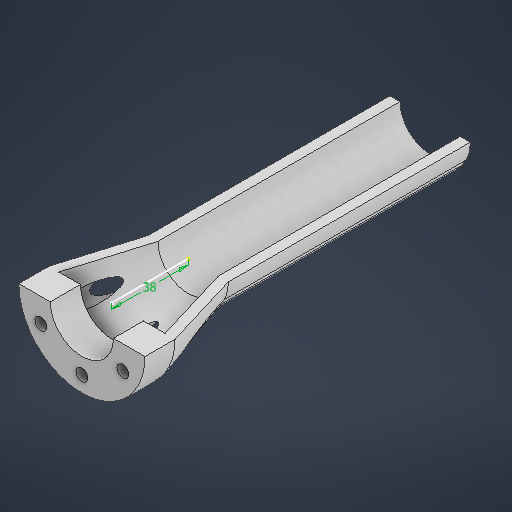
# Autodesk Inventor part: Carcasa_Part1
Saved by Autodesk Inventor 2026.1 (Build 301233020, 233B)
## iProperties
Created: 2026-01-06
Part Number: Carcasa_Part1
Material: Generic
Document SubType Name: Modeling
Designer: Marcelo
Density: 1 g/cm^3
Appearance: Default
Author: Marcelo
Autodesk Inventor part; units mm, degrees
ref_plane "YZ Plane" through (0, 0, 0) normal (1, 0, 0) x (0, 1, 0)
ref_plane "XZ Plane" through (0, 0, 0) normal (0, 1, 0) x (-1, 0, 0)
sketch "Sketch1" plane through (0, 0, 0) normal (0, 0, 1) x (1, 0, 0)
  circle A0 centre (0, 0) radius 20.05
  dimension "d0" = 40.1
  constraints: 1 centre point, 1 coincident
  measures "d0" diameter of A0
extrude "Extrusion1" add sketch "Sketch1" along normal blind 120.75
sketch "Sketch2" plane through (0, 0, 120.75) normal (0, 0, 1) x (1, 0, 0)
  circle A0 centre (0, 0) radius 20.05 projected
  arc A1 (-15.05, 0) -> (15.05, 0) centre (0, 0) ccw
  line L0 (-20.05, 0) -> (20.05, 0)
  dimension "d3" = 5
  constraints: 4 point on circle, 2 end point, 2 horizontal, 2 point on line, 1 centre point
  measures "d3" radial gap between concentric circles of A0 A1
extrude "Extrusion2" cut sketch "Sketch2" against normal blind 120.75 contours L0 A0 | A1 L0
sketch "Sketch3" plane through (0, 0, 120.75) normal (0, 0, 1) x (1, 0, 0)
  point P0 (0, 0)
sketch3d "3D Sketch1"
ref_plane "Work Plane1" through (0, 0, 158.75) normal (0, 0, 1) x (1, 0, 0)
sketch "Sketch4" plane through (0, 0, 158.75) normal (0, 0, 1) x (1, 0, 0)
  circle A0 centre (0, 0) radius 31.5
  circle A1 centre (0, 0) radius 15.75
  dimension "d7" = 63
  dimension "d8" = 31.5
  constraints: 2 centre point, 2 coincident
  measures "d7" diameter of A0
  measures "d8" diameter of A1
extrude "Extrusion3" add sketch "Sketch4" along normal blind 15
sketch "Sketch5" plane through (0, 0, 173.75) normal (0, 0, 1) x (1, 0, 0)
  line L0 (27.2798, -15.75) -> (-27.2798, 15.75)
  line L1 (0, 31.5) -> (0, -31.5)
  circle A0 centre (0, 0) radius 31.5 projected
  line L2 (27.2798, 15.75) -> (-27.2798, -15.75)
  circle A1 centre (0, 0) radius 31.5 projected
  circle A2 centre (0, 0) radius 15.75 projected
  circle A3 centre (0, 0) radius 23.625 construction
  line L3 (0, 0) -> (-31.5, 0) construction
  circle A4 centre (-20.4599, 11.8125) radius 3
  circle A5 centre (0, 23.625) radius 3
  circle A6 centre (20.4599, 11.8125) radius 3
  circle A7 centre (20.4599, -11.8125) radius 3
  circle A8 centre (0, -23.625) radius 3
  circle A9 centre (-20.4599, -11.8125) radius 3
  dimension "d14" = 60
  dimension "d15" = 60
  dimension "d16" = 7.875
  dimension "d17" = 30
  dimension "d18" = 6
  dimension "d19" = 6
  dimension "d20" = 6
  dimension "d21" = 6
  dimension "d22" = 6
  dimension "d23" = 6
  constraints: 11 point on circle, 8 end point, 7 centre point, 6 point on line, 3 midpoint, 1 coincident, 1 horizontal, 2 other
  measures "d14" angle of L1 L0
  measures "d15" angle of L0 L2
  measures "d16" radial gap between concentric circles of A3 A2
  measures "d17" angle of L3 L0
  measures "d18" diameter of A4
  measures "d19" diameter of A5
  measures "d20" diameter of A6
  measures "d21" diameter of A7
  measures "d22" diameter of A8
  measures "d23" diameter of A9
hole "Hole1" at (-20.4599, 11.8125, 173.75) direction (0, 0, -1) diameter 6 end through all
thread "Thread1" size "M6x1" class "6H" standard "ISO Metric profile" full length
pattern_circular "Circular Pattern1" count 6 over 360 about axis through (0, 0, 158.75) along (0, 0, 1) of "Hole1"
sketch "Sketch7" plane through (0, 0, 173.75) normal (0, 0, 1) x (1, 0, 0)
  circle A0 centre (0, 0) radius 31.5 projected
  line L0 (-31.5, 0) -> (31.5, 0)
  constraints: 2 end point, 2 point on circle, 1 horizontal
extrude "Extrusion4" cut sketch "Sketch7" against normal blind 15 contours L0 A0 picked at (9.2973, 4.8796)
sketch "Sketch8" plane through (0, 0, 158.75) normal (0, 0, -1) x (-1, 0, 0)
  arc A0 (-31.5, 0) -> (31.5, 0) centre (0, 0) ccw projected
  arc A1 (-26.5, 0) -> (26.5, 0) centre (0, 0) ccw
  line L0 (-15.75, 0) -> (-31.5, 0) projected
  line L1 (-31.5, 0) -> (-26.5, 0)
  line L2 (26.5, 0) -> (31.5, 0)
  dimension "d39" = 5
  constraints: 4 end point, 2 collinear, 2 point on circle, 1 centre point
  measures "d39" radial gap between concentric circles of A0 A1
loft "Loft1" add profiles "Sketch8" section 1 edges at (-17.55, 0, 120.75) (0, -20.05, 120.75) (17.55, 0, 120.75) (0, -15.05, 120.75)
sketch "Sketch10" plane through (0, 0, 158.75) normal (0, 0, -1) x (-1, 0, 0)
  circle A0 centre (-20.4599, -11.8125) radius 4
  circle A1 centre (0, -23.625) radius 4
  circle A2 centre (20.4599, -11.8125) radius 4
  line L0 (0, 0) -> (49.8293, -28.7689)
  line L1 (0, 0) -> (-50.7535, -29.3026)
  line L2 (0, 0) -> (0, -46.5464)
  line L3 (72.2557, 0) -> (-72.2557, 0) construction
  circle A3 centre (20.4599, -11.8125) radius 3 construction
  circle A4 centre (0, 0) radius 23.625 construction
  point P0 (0, -23.625)
  point P1 (-20.4599, -11.8125)
  dimension "d58" = 8
  dimension "d59" = 8
  dimension "d60" = 8
  dimension "d61" = 60
  dimension "d62" = 60
  dimension "d63" = 30
  constraints: 8 end point, 4 centre point, 3 coincident, 3 point on circle, 3 point on line, 2 midpoint, 1 horizontal
  measures "d58" diameter of A0
  measures "d59" diameter of A1
  measures "d60" diameter of A2
  measures "d61" angle of L2 L0
  measures "d62" angle of L1 L2
  measures "d63" angle of L3 L0
hole "Hole3" at (-20.4599, -11.8125, 158.75) at (0, -23.625, 158.75) at (20.4599, -11.8125, 158.75) direction (0, 0, -1) diameter 8 end through all
equation "\"d19\" = d18"
equation "\"d20\" = d18"
equation "\"d21\" = d18"
equation "\"d22\" = d18"
equation "\"d23\" = d18"
equation "\"d59\" = d58"
equation "\"d60\" = d58"
body "Solid1"
